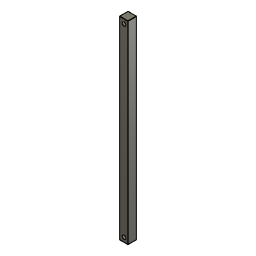
0.883.4403 - IGTE 21465_204215 Rép. 103 (Autodesk Fusion 360 design; units mm, degrees)
Autodesk Fusion 360 part; units mm, degrees
sketch "Sketch2" plane through (0, 0, 0) normal (0, 1, 0) x (1, 0, 0)
  line L0 (0, 0) -> (-28, 0)
  line L1 (-28, 0) -> (-28, 28)
  line L2 (-28, 28) -> (0, 28)
  line L3 (0, 28) -> (0, 0)
  dimension "d1" = 28
  dimension "d2" = 28
  constraint horizontal L0
  constraint vertical L1
  constraint horizontal L2
  constraint vertical L3
  constraint coincident L0.start L3.end
  measures "d1" distance of L0.start L2.end
  measures "d2" distance of L0.start L0.end
extrude "Extrude1" add sketch "Sketch2" along normal blind 635
sketch "Sketch3" plane through (0, 0, -28) normal (0, 0, -1) x (-1, 0, 0)
  line L0 (0, 0) -> (28, 0)
  line L1 (28, 0) -> (28, 635)
  line L2 (28, 635) -> (0, 635)
  line L3 (0, 635) -> (0, 0)
  circle A0 centre (13, 620) radius 6
  line L4 (28, 317.5) -> (0, 317.5) construction
  circle A1 centre (13, 15) radius 6
  dimension "d5" = 12
  dimension "d6" = 15
  dimension "d7" = 15
  constraint midpoint L1 L4.start
  constraint midpoint L3 L4.end
  constraint symmetric A0 L4 A1
  measures "d5" diameter of A0
  measures "d6" distance of L2 A0.centre
  measures "d7" distance of L1 A0.centre
extrude "Extrude2" cut sketch "Sketch3" against normal through all contours A0 | A1
fillet "Fillet1" radius 0.5 12 edges at (-28, 317.5, 0) (0, 317.5, 0) (-28, 317.5, -28) (0, 317.5, -28) (0, 635, -14) (-14, 635, -28) (-28, 635, -14) (-14, 635, 0) (-14, 0, 0) (-28, 0, -14) (0, 0, -14) (-14, 0, -28)
equation "d7 = d6"
